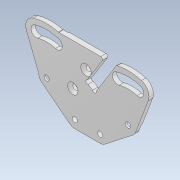
# Autodesk Inventor part: 脚中間フレーム外側
Saved by Autodesk Inventor 2020.2 (Build 242310000, 310)
## iProperties
Created: 2020-03-12
Part Number: 脚中間フレーム外側
Material: アルミニウム 2014-T4
Document SubType Name: Modeling
Designer: aoyam
Density: 2.8 g/cm^3
Appearance: サテン
Mass: 9.40624 g
Surface Area: 56.2254 cm^2
Volume: 3.35937 cm^3
Author: aoyam
Autodesk Inventor part; units mm, degrees
ref_plane "YZ Plane" through (0, 0, 0) normal (1, 0, 0) x (0, 1, 0)
ref_plane "XZ Plane" through (0, 0, 0) normal (0, 1, 0) x (-1, 0, 0)
ref_plane "XY Plane" through (0, 0, 0) normal (0, 0, 1) x (1, 0, 0)
sketch "スケッチ1" plane through (0, 0, 0) normal (0, 0, 1) x (1, 0, 0)
  circle A0 centre (-23.2, 0) radius 14.1 construction
  circle A1 centre (0, 0) radius 9.1 construction
  circle A2 centre (23.2, 0) radius 14.1 construction
  circle A3 centre (-23.2, 0) radius 1.5
  circle A4 centre (-23.2, 0) radius 4.5
  line L0 (0, 0) -> (0, 20.5296)
  line L1 (-47.939, 0) -> (0, 0)
  line L2 (0, 0) -> (0, -20)
  circle A5 centre (0, 15.5) radius 1.5
  circle A6 centre (0, 15.5) radius 4.5 construction
  circle A7 centre (0, 0) radius 11 construction
  line L3 (-38, 31) -> (38, 31)
  line L4 (38, 31) -> (38, -20)
  line L5 (38, -20) -> (-38, -20)
  line L6 (-38, -20) -> (-38, 31)
  circle A8 centre (23.2, 0) radius 4.5
  circle A9 centre (23.2, 0) radius 1.5
  arc A10 (1.5, -5.8095) -> (4.2038, 4.2812) centre (0, 0) ccw
  line L7 (-1.5, -5.8095) -> (-1.5, -11.2574)
  line L8 (1.5, -11.2574) -> (1.5, -5.8095)
  arc A11 (1.6057, 5.7812) -> (-1.6057, 5.7812) centre (0, 0) ccw
  circle A12 centre (0, 0) radius 4
  arc A13 (-4.2038, 4.2812) -> (-1.5, -5.8095) centre (0, 0) ccw
  line L9 (4.2038, 4.2812) -> (7.2283, 9.5198)
  arc A14 (7.2283, 9.5198) -> (4.6302, 11.0198) centre (7.2283, 12.5198) ccw
  line L10 (4.6302, 11.0198) -> (1.6057, 5.7812)
  line L11 (-1.6057, 5.7812) -> (-4.6302, 11.0198)
  arc A15 (-4.6302, 11.0198) -> (-7.2283, 9.5198) centre (-7.2283, 12.5198) ccw
  line L12 (-7.2283, 9.5198) -> (-4.2038, 4.2812)
  circle A16 centre (-7.2283, 12.5198) radius 1.5
  circle A17 centre (7.2283, 12.5198) radius 1.5
  circle A18 centre (-7.2283, -12.5198) radius 1.5
  circle A19 centre (7.2283, -12.5198) radius 1.5
  circle A20 centre (-7.2283, -12.5198) radius 4.5
  circle A21 centre (7.2283, -12.5198) radius 4.5
  line L13 (-25.9762, -3.5416) -> (-10.0045, -16.0614)
  line L14 (-7.2283, -17.0198) -> (7.2283, -17.0198)
  line L15 (10.0045, -16.0614) -> (25.9762, -3.5416)
  line L16 (23.2, 0) -> (38, 0)
  circle A22 centre (7.2283, -12.5198) radius 1.5
  circle A23 centre (-7.2283, -12.5198) radius 1.5
  arc A24 (-18.134, 17.0975) -> (-28.266, 17.0975) centre (-23.2, 0) ccw
  arc A25 (-29.9847, 22.8983) -> (-28.266, 17.0975) centre (-29.1254, 19.9979) ccw
  arc A26 (-16.4153, 22.8983) -> (-29.9847, 22.8983) centre (-23.2, 0) ccw
  arc A27 (-18.134, 17.0975) -> (-16.4153, 22.8983) centre (-17.2746, 19.9979) ccw
  circle A28 centre (0, 15.5) radius 1.5
  arc A29 (28.266, 17.0975) -> (18.134, 17.0975) centre (23.2, 0) ccw
  arc A30 (16.4153, 22.8983) -> (18.134, 17.0975) centre (17.2746, 19.9979) ccw
  arc A31 (29.9847, 22.8983) -> (16.4153, 22.8983) centre (23.2, 0) ccw
  arc A32 (28.266, 17.0975) -> (29.9847, 22.8983) centre (29.1254, 19.9979) ccw
  line L17 (-34, 26) -> (34, 26)
  line L18 (-29.1254, 19.9979) -> (-23.2, 0)
  line L19 (-23.2, 0) -> (-17.2746, 19.9979)
  circle A33 centre (-9.2601, 26) radius 1.25
  circle A34 centre (-23.2, 0) radius 4.5
  circle A35 centre (23.2, 0) radius 4.5
  arc A36 (-18.9863, 14.2211) -> (-27.4137, 14.2211) centre (-23.2, 0) ccw
  arc A37 (-18.9863, 14.2211) -> (-15.563, 25.7747) centre (-17.2746, 19.9979) ccw
  arc A38 (-15.563, 25.7747) -> (-30.837, 25.7747) centre (-23.2, 0) ccw
  arc A39 (-30.837, 25.7747) -> (-27.4137, 14.2211) centre (-29.1254, 19.9979) ccw
  circle A40 centre (-9.2601, 26) radius 4.25
  arc A41 (27.4137, 14.2211) -> (18.9863, 14.2211) centre (23.2, 0) ccw
  arc A42 (27.4137, 14.2211) -> (30.837, 25.7747) centre (29.1254, 19.9979) ccw
  arc A43 (30.837, 25.7747) -> (15.563, 25.7747) centre (23.2, 0) ccw
  arc A44 (15.563, 25.7747) -> (18.9863, 14.2211) centre (17.2746, 19.9979) ccw
  line L20 (-27.7, 0) -> (-34.7286, 17.7833)
  line L21 (-23.2, 26.8823) -> (-10.295, 30.1221)
  line L22 (-8.2253, 30.1221) -> (23.2, 26.8823)
  line L23 (34.9021, 18.2863) -> (27.4137, -1.5794)
  point P0 (-27.7, 0)
  point P1 (27.7, 0)
  point P2 (-38, 0)
  point P3 (28.0091, 0)
  point P4 (34.5946, 17.4704)
  point P5 (-27.7, 0)
  point P6 (27.4137, -1.5794)
  point P7 (16.3694, 26)
  point P8 (-16.3694, 26)
  dimension "d55" = 9
  dimension "d56" = 9
  dimension "d0" = 28.2
  dimension "d1" = 28.2
  dimension "d2" = 18.2
  dimension "d3" = 3
  dimension "d4" = 3
  dimension "d5" = 3
  dimension "d6" = 3
  dimension "d7" = 22
  dimension "d8" = 38
  dimension "d11" = 31
  dimension "d14" = 20
  dimension "d15" = 3
  dimension "d16" = 3
  dimension "d17" = 38
  dimension "d44" = 3
  dimension "d45" = 3
  dimension "d51" = 33.009
  dimension "d52" = 2.5
  dimension "d53" = 14
  dimension "d54" = 10.5
  dimension "d57" = 3
  dimension "d58" = 3
  dimension "d59" = 3
  constraints: 52 point on circle, 48 end point, 41 centre point, 8 tangent, 6 coincident, 5 horizontal, 4 point on line, 3 symmetric about line, 3 vertical, 2 parallel, 2 perpendicular, 1 horizontal alignment, 46 other
  measures "d0" diameter of A2
  measures "d1" diameter of A0
  measures "d2" diameter of A1
  measures "d3" diameter of A3
  measures "d4" diameter of A3
  measures "d5" diameter of A5
  measures "d6" radial gap between concentric circles of A5 A6
  measures "d7" diameter of A7
  measures "d8" distance between parallel lines of L6 L0
  measures "d11" distance between parallel lines of L1 L3
  measures "d14" distance between parallel lines of L5 L1
  measures "d15" diameter of A16
  measures "d16" diameter of A17
  measures "d17" distance between parallel lines of L4 L0
  measures "d44" radial gap between concentric circles of A20 A18
  measures "d45" radial gap between concentric circles of A19 A21
  measures "d51" angle of L19 L18
  measures "d52" diameter of A33
  measures "d53" distance of A28.centre A33.centre
  measures "d54" distance from line of A28.centre L17
  measures "d57" radial gap between concentric circles of A24 A36
  measures "d58" radial gap between concentric circles of A33 A40
  measures "d59" radial gap between concentric circles of A30 A44
extrude "押し出し1" add sketch "スケッチ1" along normal blind 3 contours L1 A4 A3 | A3 L19 A4 L1 | A3 L18 A4 L19 | L1 A4 L18 A3 | L1 A12 L2 L14 A20 L13 A4 | A4 L19 A37 A40 L17 A43 A44 A41 A42 L23 L16 A8 L15 A21 L14 L2 A12 L0 A11 L11 A15 L12 A13 L1 | A4 L18 A36 L19 | L20 A39 L18 A4 | A13 L12 A15 L11 A11 L0 A12 L1 | A36 L18 A24 L19 | L19 A27 A26 A25 L18 A39 A38 L17 A37 A40 | A20 | A12 L0 L1 | L1 L2 A12 | A40 A37 | A37 A40 L17 A33 | L0 A12 L2 | A37 A38 L17 A40 | A38 L17 | A33 L17 | A43 L17 | L17 A43 A42 L23 A41 A44 | A21 | L23 A8 L16 | A8 | L23 A42 | A5 L0 | L0 A5 | A16 | A17 picked at (-9.1528, 25.1164)
sketch "スケッチ3" plane through (0, 0, 3) normal (0, 0, 1) x (1, 0, 0)
  circle A0 centre (7.2283, -12.5198) radius 1.5
  circle A1 centre (-7.2283, -12.5198) radius 1.5
  arc A2 (-18.134, 17.0975) -> (-28.266, 17.0975) centre (-23.2, 0) ccw
  arc A3 (-29.9847, 22.8983) -> (-28.266, 17.0975) centre (-29.1254, 19.9979) ccw
  arc A4 (-16.4153, 22.8983) -> (-29.9847, 22.8983) centre (-23.2, 0) ccw
  arc A5 (-18.134, 17.0975) -> (-16.4153, 22.8983) centre (-17.2746, 19.9979) ccw
  circle A6 centre (0, 15.5) radius 1.5
  arc A7 (28.266, 17.0975) -> (18.134, 17.0975) centre (23.2, 0) ccw
  arc A8 (16.4153, 22.8983) -> (18.134, 17.0975) centre (17.2746, 19.9979) ccw
  arc A9 (29.9847, 22.8983) -> (16.4153, 22.8983) centre (23.2, 0) ccw
  arc A10 (28.266, 17.0975) -> (29.9847, 22.8983) centre (29.1254, 19.9979) ccw
  line L0 (-34, 26) -> (34, 26)
  line L1 (-29.1254, 19.9979) -> (-23.2, 0)
  line L2 (-23.2, 0) -> (-17.2746, 19.9979)
  circle A11 centre (-9.2601, 26) radius 1.25
  circle A12 centre (-23.2, 0) radius 4.5
  circle A13 centre (23.2, 0) radius 4.5
  arc A14 (-18.9863, 14.2211) -> (-27.4137, 14.2211) centre (-23.2, 0) ccw
  arc A15 (-18.9863, 14.2211) -> (-15.563, 25.7747) centre (-17.2746, 19.9979) ccw
  arc A16 (-15.563, 25.7747) -> (-30.837, 25.7747) centre (-23.2, 0) ccw
  arc A17 (-30.837, 25.7747) -> (-27.4137, 14.2211) centre (-29.1254, 19.9979) ccw
  circle A18 centre (-9.2601, 26) radius 4.25
  arc A19 (27.4137, 14.2211) -> (18.9863, 14.2211) centre (23.2, 0) ccw
  arc A20 (27.4137, 14.2211) -> (30.837, 25.7747) centre (29.1254, 19.9979) ccw
  arc A21 (30.837, 25.7747) -> (15.563, 25.7747) centre (23.2, 0) ccw
  arc A22 (15.563, 25.7747) -> (18.9863, 14.2211) centre (17.2746, 19.9979) ccw
  line L3 (-27.7, 0) -> (-34.7286, 17.7833)
  line L4 (-23.2, 26.8823) -> (-10.295, 30.1221)
  line L5 (-8.2253, 30.1221) -> (23.2, 26.8823)
  line L6 (34.9021, 18.2863) -> (27.4137, -1.5794)
  point P0 (0, 0)
  point P1 (0, 0)
  dimension "d46" = 9
  dimension "d47" = 9
  dimension "d38" = 33.009
  dimension "d39" = 2.5
  dimension "d40" = 14
  dimension "d41" = 10.5
  dimension "d48" = 3
  dimension "d49" = 3
  dimension "d50" = 3
  constraints: 38 point on circle, 21 centre point, 14 end point, 2 tangent, 1 coincident, 1 horizontal, 1 horizontal alignment, 1 point on line, 32 other
  measures "d38" angle of L2 L1
  measures "d39" diameter of A11
  measures "d40" distance of A6.centre A11.centre
  measures "d41" distance from line of A6.centre L0
  measures "d48" radial gap between concentric circles of A2 A14
  measures "d49" radial gap between concentric circles of A11 A18
  measures "d50" radial gap between concentric circles of A8 A22
sketch "スケッチ5" plane through (0, 0, 0) normal (0, 0, -1) x (-1, 0, 0)
  circle A0 centre (-23.2, 0) radius 1.5 projected
  circle A1 centre (23.2, 0) radius 1.5 projected
  circle A2 centre (-23.2, 0) radius 3
  circle A3 centre (23.2, 0) radius 3
  point P0 (0, 0)
  dimension "d25" = 6
  dimension "d26" = 6
  constraints: 2 centre point, 2 coincident
  measures "d25" diameter of A2
  measures "d26" diameter of A3
extrude "押し出し4" cut sketch "スケッチ5" against normal blind 2
sketch "スケッチ6" plane through (0, 0, 0) normal (0, 0, -1) x (-1, 0, 0)
  circle A0 centre (-7.2283, -12.5198) radius 1.5 projected
  circle A1 centre (7.2283, -12.5198) radius 1.5 projected
  circle A2 centre (-7.2283, -12.5198) radius 3
  circle A3 centre (7.2283, -12.5198) radius 3
  point P0 (0, 0)
  dimension "d32" = 6
  dimension "d33" = 6
  constraints: 2 centre point, 2 coincident
  measures "d32" diameter of A2
  measures "d33" diameter of A3
extrude "押し出し5" cut sketch "スケッチ6" against normal blind 0.5
sketch "スケッチ9" plane through (0, 0, 3) normal (0, 0, 1) x (1, 0, 0)
  line L0 (27.4137, -1.5794) -> (34.5946, 17.4704) projected
  arc A0 (34.5946, 17.4704) -> (30.837, 25.7747) centre (29.1254, 19.9979) ccw projected
  arc A1 (30.837, 25.7747) -> (16.3694, 26) centre (23.2, 0) ccw projected
  arc A2 (-16.3694, 26) -> (-30.837, 25.7747) centre (-23.2, 0) ccw projected
  arc A3 (-30.837, 25.7747) -> (-34.7286, 17.7833) centre (-29.1254, 19.9979) ccw projected
  line L1 (-34.7286, 17.7833) -> (-27.7, 0) projected
  arc A4 (-27.7, 0) -> (-25.9762, -3.5416) centre (-23.2, 0) ccw projected
  line L2 (-25.9762, -3.5416) -> (-10.0045, -16.0614) projected
  arc A5 (-10.0045, -16.0614) -> (-7.2283, -17.0198) centre (-7.2283, -12.5198) ccw projected
  line L3 (-7.2283, -17.0198) -> (7.2283, -17.0198) projected
  arc A6 (7.2283, -17.0198) -> (10.0045, -16.0614) centre (7.2283, -12.5198) ccw projected
  line L4 (10.0045, -16.0614) -> (25.9762, -3.5416) projected
  arc A7 (25.9762, -3.5416) -> (27.4137, -1.5794) centre (23.2, 0) ccw projected
  circle A8 centre (-7.2283, -12.5198) radius 1.5 projected
  circle A9 centre (23.2, 0) radius 1.5 projected
  circle A10 centre (-23.2, 0) radius 1.5 projected
  circle A11 centre (7.2283, -12.5198) radius 1.5 projected
  arc A12 (28.266, 17.0975) -> (29.9847, 22.8983) centre (29.1254, 19.9979) ccw projected
  arc A13 (28.266, 17.0975) -> (18.134, 17.0975) centre (23.2, 0) ccw projected
  arc A14 (16.4153, 22.8983) -> (18.134, 17.0975) centre (17.2746, 19.9979) ccw projected
  arc A15 (29.9847, 22.8983) -> (16.4153, 22.8983) centre (23.2, 0) ccw projected
  arc A16 (-29.9847, 22.8983) -> (-28.266, 17.0975) centre (-29.1254, 19.9979) ccw projected
  arc A17 (-16.4153, 22.8983) -> (-29.9847, 22.8983) centre (-23.2, 0) ccw projected
  arc A18 (-18.134, 17.0975) -> (-16.4153, 22.8983) centre (-17.2746, 19.9979) ccw projected
  arc A19 (-18.134, 17.0975) -> (-28.266, 17.0975) centre (-23.2, 0) ccw projected
  line L5 (16.3694, 26) -> (-16.3694, 26) projected
  point P0 (0, 0)
sketch "翼" plane through (0, 0, 3) normal (0, 0, 1) x (1, 0, 0)
  arc A0 (-18.1381, 17.1031) -> (-16.4194, 22.9038) centre (-17.2788, 20.0034) ccw
  arc A1 (28.2619, 17.1031) -> (29.9806, 22.9038) centre (29.1212, 20.0034) ccw
  line L0 (27.4137, -1.5794) -> (34.5946, 17.4704) projected
  arc A2 (34.5946, 17.4704) -> (30.837, 25.7747) centre (29.1254, 19.9979) ccw projected
  arc A3 (30.837, 25.7747) -> (16.3694, 26) centre (23.2, 0) ccw projected
  line L1 (16.3694, 26) -> (-16.3694, 26) projected
  arc A4 (-16.3694, 26) -> (-30.837, 25.7747) centre (-23.2, 0) ccw projected
  arc A5 (-30.837, 25.7747) -> (-34.7286, 17.7833) centre (-29.1254, 19.9979) ccw projected
  line L2 (-34.7286, 17.7833) -> (-27.7, 0) projected
  arc A6 (-27.7, 0) -> (-25.9762, -3.5416) centre (-23.2, 0) ccw projected
  line L3 (-25.9762, -3.5416) -> (-10.0045, -16.0614) projected
  arc A7 (-10.0045, -16.0614) -> (-7.2283, -17.0198) centre (-7.2283, -12.5198) ccw projected
  line L4 (-7.2283, -17.0198) -> (7.2283, -17.0198) projected
  arc A8 (7.2283, -17.0198) -> (10.0045, -16.0614) centre (7.2283, -12.5198) ccw projected
  line L5 (10.0045, -16.0614) -> (25.9762, -3.5416) projected
  arc A9 (25.9762, -3.5416) -> (27.4137, -1.5794) centre (23.2, 0) ccw projected
  arc A10 (28.266, 17.0975) -> (18.134, 17.0975) centre (23.2, 0) ccw projected
  arc A11 (16.4153, 22.8983) -> (18.134, 17.0975) centre (17.2746, 19.9979) ccw projected
  arc A12 (29.9847, 22.8983) -> (16.4153, 22.8983) centre (23.2, 0) ccw projected
  arc A13 (28.266, 17.0975) -> (29.9847, 22.8983) centre (29.1254, 19.9979) ccw projected
  arc A14 (-29.9847, 22.8983) -> (-28.266, 17.0975) centre (-29.1254, 19.9979) ccw projected
  arc A15 (-16.4153, 22.8983) -> (-29.9847, 22.8983) centre (-23.2, 0) ccw projected
  arc A16 (-18.134, 17.0975) -> (-16.4153, 22.8983) centre (-17.2746, 19.9979) ccw projected
  arc A17 (-18.134, 17.0975) -> (-28.266, 17.0975) centre (-23.2, 0) ccw projected
  circle A18 centre (-23.2, 0) radius 1.5 projected
  circle A19 centre (7.2283, -12.5198) radius 1.5 projected
  circle A20 centre (23.2, 0) radius 1.5 projected
  circle A21 centre (-7.2283, -12.5198) radius 1.5 projected
  line L6 (0.0889, 10.0467) -> (15.7158, 35.055)
  line L7 (15.7158, 35.055) -> (19.9561, 32.4054)
  line L8 (19.9561, 32.4054) -> (4.3292, 7.3971)
  line L9 (4.3292, 7.3971) -> (0.0889, 10.0467)
  line L10 (15.5568, 35.744) -> (-0.865, 9.4636)
  line L11 (-0.865, 9.4636) -> (4.2233, 6.2841)
  line L12 (4.2233, 6.2841) -> (20.6451, 32.5644)
  line L13 (20.6451, 32.5644) -> (15.5568, 35.744)
  line L14 (-11.2804, 3.1744) -> (-0.2027, 20.9024)
  circle A22 centre (-0.7595, 15.2936) radius 1.5
  circle A23 centre (-8.2799, 2.315) radius 1.5
  circle A24 centre (0.1581, 9.6998) radius 1.05
  circle A25 centre (3.9871, 7.3072) radius 1.05
  line L15 (0.1581, 9.6998) -> (-0.865, 9.4636)
  line L16 (4.2233, 6.2841) -> (3.9871, 7.3072)
  point P0 (0, 0)
  point P1 (4.3292, 7.3971)
  point P2 (0.3943, 8.6767)
  point P3 (-0.0781, 10.7229)
  point P4 (5.0102, 7.5434)
  point P5 (2.964, 7.071)
  dimension "d279" = 2.1
  dimension "d280" = 2.1
  dimension "d250" = 5
  dimension "d251" = 58
  dimension "d252" = 0.5
  dimension "d253" = 6
  dimension "d254" = 3
  dimension "d255" = 3
  dimension "d256" = 3
  dimension "d257" = 3
  dimension "d258" = 15
  dimension "d259" = 4
  dimension "d277" = 0.5
  dimension "d278" = 1
  dimension "d282" = 45
  dimension "d283" = 45
  constraints: 22 end point, 4 centre point, 4 point on circle, 2 parallel, 2 perpendicular, 1 coincident, 17 other
  measures "d250" distance between parallel lines of L8 L6
  measures "d251" angle of L1 L8
  measures "d252" distance between parallel lines of L6 L10
  measures "d253" distance between parallel lines of L14 L6
  measures "d254" diameter of A22
  measures "d255" diameter of A23
  measures "d256" distance from line of L10 A22.centre
  measures "d257" distance from line of L14 A23.centre
  measures "d258" distance of A22.centre A23.centre
  measures "d259" distance from line of L9 A22.centre
  measures "d277" distance between parallel lines of L12 L8
  measures "d278" distance between parallel lines of L11 L9
  measures "d282" angle of L15 L10
  measures "d283" angle of L11 L16
extrude "押し出し13" cut sketch "翼" against normal blind 10 contours L12 A25 L8 L1 A3 | A3 L1 L8 L7 L6 L10 L13 L12 | A25 L12 | L12 L11 A25 L9 L8 | L8 A25 L9 A24 L6 L1 | L1 L6 L7 L8 | A25 L11 | L8 L9 A25 | L6 A24 L10 L1 | L11 A24 L9 A25 | A24 L9 L6 | L6 L9 A24 L11 L10 | A24 L11 | L10 A24 | A22 | A23
sketch "スケッチ10" plane through (0, 0, 0) normal (0, 0, -1) x (-1, 0, 0)
  arc A0 (-11.2521, 18.8307) -> (-13.5147, 24.8231) centre (-17.1301, 20.0347) ccw
  line L0 (-31.1595, 38.1455) -> (-13.5147, 24.8231)
  line L1 (-11.2521, 18.8307) -> (-15.418, -1.5082)
  arc A1 (-25.2739, -7.6441) -> (-15.418, -1.5082) centre (-23.2553, 0.0971) ccw
  arc A2 (-16.4706, 22.9953) -> (-30.04, 22.9953) centre (-23.2553, 0.0971) ccw
  arc A3 (-30.04, 22.9953) -> (-28.3213, 17.1946) centre (-29.1807, 20.095) ccw
  arc A4 (-18.1893, 17.1946) -> (-28.3213, 17.1946) centre (-23.2553, 0.0971) ccw
  arc A5 (-18.1893, 17.1946) -> (-16.4706, 22.9953) centre (-17.3299, 20.095) ccw
  line L2 (-30.5569, 38.9436) -> (-12.9121, 25.6211)
  arc A6 (-10.2725, 18.6301) -> (-12.9121, 25.6211) centre (-17.1301, 20.0347) ccw
  line L3 (-10.2725, 18.6301) -> (-14.4383, -1.7088)
  arc A7 (-25.5262, -8.6117) -> (-14.4383, -1.7088) centre (-23.2553, 0.0971) ccw
  circle A8 centre (-7.2283, -12.5198) radius 3 projected
  line L4 (-27.4137, -1.5794) -> (-34.5946, 17.4704) projected
  line L5 (-10.0045, -16.0614) -> (-25.9762, -3.5416) projected
  arc A9 (-10.0045, -16.0614) -> (-7.2283, -17.0198) centre (-7.2283, -12.5198) ccw projected
  line L6 (7.2283, -17.0198) -> (-7.2283, -17.0198) projected
  line L7 (25.9762, -3.5416) -> (10.0045, -16.0614) projected
  line L8 (34.7286, 17.7833) -> (27.7, 0) projected
  arc A10 (34.7286, 17.7833) -> (30.837, 25.7747) centre (29.1254, 19.9979) ccw projected
  arc A11 (30.837, 25.7747) -> (16.3694, 26) centre (23.2, 0) ccw projected
  line L9 (-9.6042, 26) -> (16.3694, 26) projected
  arc A12 (-16.7719, 26.1024) -> (-30.837, 25.7747) centre (-23.2, 0) ccw projected
  arc A13 (-30.837, 25.7747) -> (-34.5946, 17.4704) centre (-29.1254, 19.9979) ccw projected
  arc A14 (-18.134, 17.0975) -> (-28.266, 17.0975) centre (-23.2, 0) ccw projected
  arc A15 (-29.9847, 22.8983) -> (-28.266, 17.0975) centre (-29.1254, 19.9979) ccw projected
  arc A16 (-16.4153, 22.8983) -> (-29.9847, 22.8983) centre (-23.2, 0) ccw projected
  arc A17 (-18.134, 17.0975) -> (-16.4153, 22.8983) centre (-17.2746, 19.9979) ccw projected
  arc A18 (28.266, 17.0975) -> (29.9847, 22.8983) centre (29.1254, 19.9979) ccw projected
  arc A19 (28.266, 17.0975) -> (18.134, 17.0975) centre (23.2, 0) ccw projected
  arc A20 (16.4153, 22.8983) -> (18.134, 17.0975) centre (17.2746, 19.9979) ccw projected
  arc A21 (29.9847, 22.8983) -> (16.4153, 22.8983) centre (23.2, 0) ccw projected
  line L10 (3.3826, 0) -> (3.3826, 26)
  line L11 (37.3221, 38.9436) -> (19.6773, 25.6211)
  arc A22 (19.6773, 25.6211) -> (17.0377, 18.6301) centre (23.8953, 20.0347) ccw
  line L12 (17.0377, 18.6301) -> (21.2036, -1.7088)
  arc A23 (21.2036, -1.7088) -> (32.2915, -8.6117) centre (30.0205, 0.0971) ccw
  arc A24 (-27.4137, -1.5794) -> (-25.9762, -3.5416) centre (-23.2, 0) ccw projected
  arc A25 (7.2283, -17.0198) -> (10.0045, -16.0614) centre (7.2283, -12.5198) ccw projected
  arc A26 (25.9762, -3.5416) -> (27.7, 0) centre (23.2, 0) ccw projected
  line L13 (-0.6699, 9.1236) -> (-3.2296, 7.5019) projected
  line L14 (-5.2787, 7.9615) -> (-16.7719, 26.1024) projected
  line L15 (-9.6042, 26) -> (-0.2103, 11.1726) projected
  arc A27 (-0.6699, 9.1236) -> (-0.2103, 11.1726) centre (-0.4401, 10.1481) ccw projected
  arc A28 (-5.2787, 7.9615) -> (-3.2296, 7.5019) centre (-4.2541, 7.7317) ccw projected
  point P0 (13.4139, 26)
  point P1 (23.1707, -5.7407)
  point P2 (-19.9427, -8.2711)
  point P3 (-13.4139, 26)
  point P4 (-31.781, 18.5494)
  point P5 (-14.6743, 21.5435)
  point P6 (21.2542, 26.8118)
  point P7 (-10.7037, 16.5244)
  point P8 (17.3768, 16.9746)
  point P9 (17.6686, 23.2329)
  dimension "d177" = 1
  constraints: 20 point on circle, 14 end point, 10 centre point, 7 symmetric about line, 1 midpoint, 9 other
  measures "d177" distance between parallel lines of L0 L2
sketch "スケッチ13" plane through (0, 0, 0.5) normal (0, 0, -1) x (-1, 0, 0)
  circle A0 centre (-7.2283, -12.5198) radius 1.5 projected
  circle A1 centre (7.2283, -12.5198) radius 1.5 projected
  arc A2 (30.1268, 23.3777) -> (16.7004, 23.5) centre (23.2, 0) ccw
  arc A3 (32.4036, 18.7022) -> (30.1268, 23.3777) centre (29.1254, 19.9979) ccw
  line L0 (32.4036, 18.7022) -> (27.8387, 7.1525)
  arc A4 (27.8387, 7.1525) -> (17.9117, -6.6865) centre (23.2, 0) ccw
  line L1 (17.9117, -6.6865) -> (8.4622, -14.0938)
  arc A5 (7.2283, -14.5198) -> (8.4622, -14.0938) centre (7.2283, -12.5198) ccw
  line L2 (7.2283, -14.5198) -> (-7.2283, -14.5198)
  arc A6 (-8.4622, -14.0938) -> (-7.2283, -14.5198) centre (-7.2283, -12.5198) ccw
  line L3 (-8.4622, -14.0938) -> (-17.9117, -6.6865)
  arc A7 (-17.9117, -6.6865) -> (-27.9945, 7.049) centre (-23.2, 0) ccw
  line L4 (-27.9945, 7.049) -> (-32.2915, 18.4482)
  arc A8 (-30.1268, 23.3777) -> (-32.2915, 18.4482) centre (-29.1254, 19.9979) ccw
  arc A9 (-18.3304, 23.8911) -> (-30.1268, 23.3777) centre (-23.2, 0) ccw
  line L5 (-18.3304, 23.8911) -> (-5.2578, 3.2573)
  line L6 (-5.2578, 3.2573) -> (4.0342, 9.1444)
  line L7 (4.0342, 9.1444) -> (-5.0608, 23.5)
  line L8 (-5.0608, 23.5) -> (16.7004, 23.5)
  line L9 (-23.2, 0) -> (-9.8054, 10.4352) construction
  line L10 (-22.4318, -0.9861) -> (-9.0372, 9.4491)
  line L11 (-10.5736, 11.4212) -> (-23.9682, 0.9861)
  arc A10 (-23.9682, 0.9861) -> (-22.4318, -0.9861) centre (-23.2, 0) ccw
  arc A11 (-9.0372, 9.4491) -> (-10.5736, 11.4212) centre (-9.8054, 10.4352) ccw
  line L12 (-7.2283, -12.5198) -> (-5.2578, 3.2573) construction
  line L13 (-5.9879, -12.6747) -> (-4.0175, 3.1024)
  line L14 (-6.4982, 3.4123) -> (-8.4687, -12.3649)
  arc A12 (-8.4687, -12.3649) -> (-5.9879, -12.6747) centre (-7.2283, -12.5198) ccw
  arc A13 (-4.0175, 3.1024) -> (-6.4982, 3.4123) centre (-5.2578, 3.2573) ccw
  line L15 (4.0342, 9.1444) -> (23.2, 0) construction
  line L16 (3.496, 8.0162) -> (22.6617, -1.1282)
  line L17 (23.7383, 1.1282) -> (4.5725, 10.2726)
  arc A14 (4.5725, 10.2726) -> (3.496, 8.0162) centre (4.0342, 9.1444) ccw
  arc A15 (22.6617, -1.1282) -> (23.7383, 1.1282) centre (23.2, 0) ccw
  line L18 (17.2746, 19.9979) -> (4.0342, 9.1444) construction
  line L19 (16.4822, 20.9646) -> (3.2418, 10.1111)
  line L20 (4.8267, 8.1777) -> (18.0671, 19.0312)
  arc A16 (18.0671, 19.0312) -> (16.4822, 20.9646) centre (17.2746, 19.9979) ccw
  arc A17 (3.2418, 10.1111) -> (4.8267, 8.1777) centre (4.0342, 9.1444) ccw
  line L21 (7.2283, -12.6747) -> (0.2333, 6.7363) construction
  line L22 (8.4043, -12.2509) -> (1.4092, 7.16)
  line L23 (-0.9427, 6.3125) -> (6.0523, -13.0985)
  arc A18 (6.0523, -13.0985) -> (8.4043, -12.2509) centre (7.2283, -12.6747) ccw
  arc A19 (1.4092, 7.16) -> (-0.9427, 6.3125) centre (0.2333, 6.7363) ccw
  circle A20 centre (-7.2283, -12.5198) radius 4
  circle A21 centre (7.2283, -12.5198) radius 4
  arc A22 (-30.695, 25.2953) -> (-27.5558, 14.7005) centre (-29.1254, 19.9979) ccw
  arc A23 (-15.705, 25.2953) -> (-30.695, 25.2953) centre (-23.2, 0) ccw
  arc A24 (-18.8442, 14.7005) -> (-15.705, 25.2953) centre (-17.2746, 19.9979) ccw
  arc A25 (-18.8442, 14.7005) -> (-27.5558, 14.7005) centre (-23.2, 0) ccw
  arc A26 (27.5558, 14.7005) -> (18.8442, 14.7005) centre (23.2, 0) ccw
  arc A27 (27.5558, 14.7005) -> (30.695, 25.2953) centre (29.1254, 19.9979) ccw
  arc A28 (30.695, 25.2953) -> (15.705, 25.2953) centre (23.2, 0) ccw
  arc A29 (15.705, 25.2953) -> (18.8442, 14.7005) centre (17.2746, 19.9979) ccw
  point P0 (0, 0)
  point P1 (-16.5027, 5.2176)
  point P2 (-6.2431, -4.6312)
  point P3 (13.6171, 4.5722)
  point P4 (10.6544, 14.5711)
  point P5 (3.7308, -2.9692)
  point P6 (12.3201, 17.5528)
  point P7 (13.0014, 23.5)
  point P8 (3.3603, 10.2082)
  point P9 (13.905, 15.6194)
  point P10 (6.3485, 9.4252)
  point P11 (16.1273, 4.7595)
  point P12 (30.8398, 14.7456)
  point P13 (7.061, -8.5233)
  point P14 (11.1885, -11.9567)
  point P15 (15.0508, 2.5032)
  point P16 (2.9783, 8.4754)
  point P17 (1.2892, 7.4052)
  point P18 (3.7642, -14.5198)
  point P19 (4.7207, -9.4034)
  point P20 (-0.8485, 6.0509)
  point P21 (-4.2019, 3.9263)
  point P22 (-5.517, -8.9043)
  point P23 (-3.7642, -14.5198)
  point P24 (-11.1885, -11.9567)
  point P25 (-7.9978, -8.5945)
  point P26 (-5.9268, 4.3133)
  point P27 (-9.1332, 9.3742)
  point P28 (-15.7794, 4.1965)
  point P29 (-30.9038, 14.767)
  point P30 (-17.3158, 6.1686)
  point P31 (-10.4743, 11.4911)
  point P32 (-13.3807, 16.0784)
  dimension "d189" = 2.5
  dimension "d190" = 2.5
  dimension "d191" = 2.5
  dimension "d192" = 2.5
  dimension "d193" = 2.5
  dimension "d194" = 2.5
  dimension "d195" = 2.5
  constraints: 58 end point, 52 point on circle, 28 centre point, 20 tangent, 5 midpoint, 5 parallel, 2 point on line
  measures "d189" diameter of A11
  measures "d190" diameter of A13
  measures "d191" diameter of A15
  measures "d192" diameter of A17
  measures "d193" diameter of A19
  measures "d194" radial gap between concentric circles of A0 A20
  measures "d195" radial gap between concentric circles of A1 A21
sketch "スケッチ20" plane through (0, 0, 0) normal (0, 0, -1) x (-1, 0, 0)
  arc A0 (28.266, 17.0975) -> (29.9847, 22.8983) centre (29.1254, 19.9979) ccw projected
  arc A1 (28.266, 17.0975) -> (18.134, 17.0975) centre (23.2, 0) ccw projected
  arc A2 (16.4153, 22.8983) -> (18.134, 17.0975) centre (17.2746, 19.9979) ccw projected
  arc A3 (29.9847, 22.8983) -> (16.4153, 22.8983) centre (23.2, 0) ccw projected
  arc A4 (-18.134, 17.0975) -> (-28.266, 17.0975) centre (-23.2, 0) ccw projected
  arc A5 (-29.9847, 22.8983) -> (-28.266, 17.0975) centre (-29.1254, 19.9979) ccw projected
  arc A6 (-16.4153, 22.8983) -> (-29.9847, 22.8983) centre (-23.2, 0) ccw projected
  arc A7 (-18.134, 17.0975) -> (-16.4153, 22.8983) centre (-17.2746, 19.9979) ccw projected
  line L0 (-9.4681, 26) -> (0.0781, 10.7229) projected
  line L1 (-0.3943, 8.6767) -> (-2.964, 7.071) projected
  line L2 (-5.0102, 7.5434) -> (-16.5766, 26.0535) projected
  arc A8 (-16.5766, 26.0535) -> (-30.837, 25.7747) centre (-23.2, 0) ccw projected
  arc A9 (-30.837, 25.7747) -> (-34.5946, 17.4704) centre (-29.1254, 19.9979) ccw projected
  line L3 (-27.4137, -1.5794) -> (-34.5946, 17.4704) projected
  arc A10 (-27.4137, -1.5794) -> (-25.9762, -3.5416) centre (-23.2, 0) ccw projected
  line L4 (-10.0045, -16.0614) -> (-25.9762, -3.5416) projected
  arc A11 (-10.0045, -16.0614) -> (-7.2283, -17.0198) centre (-7.2283, -12.5198) ccw projected
  line L5 (7.2283, -17.0198) -> (-7.2283, -17.0198) projected
  arc A12 (7.2283, -17.0198) -> (10.0045, -16.0614) centre (7.2283, -12.5198) ccw projected
  line L6 (25.9762, -3.5416) -> (10.0045, -16.0614) projected
  arc A13 (25.9762, -3.5416) -> (27.7, 0) centre (23.2, 0) ccw projected
  line L7 (34.7286, 17.7833) -> (27.7, 0) projected
  arc A14 (34.7286, 17.7833) -> (30.837, 25.7747) centre (29.1254, 19.9979) ccw projected
  arc A15 (30.837, 25.7747) -> (16.3694, 26) centre (23.2, 0) ccw projected
  line L8 (-9.4681, 26) -> (16.3694, 26) projected
  circle A16 centre (-23.2, 0) radius 3 projected
  circle A17 centre (23.2, 0) radius 3 projected
  circle A18 centre (-7.2283, -12.5198) radius 3 projected
  circle A19 centre (7.2283, -12.5198) radius 3 projected
  circle A20 centre (0.7595, 15.2936) radius 1.5 projected
  circle A21 centre (8.2799, 2.315) radius 1.5 projected
  arc A22 (30.1268, 23.3777) -> (16.7004, 23.5) centre (23.2, 0) ccw
  arc A23 (32.4036, 18.7022) -> (30.1268, 23.3777) centre (29.1254, 19.9979) ccw
  line L9 (32.4036, 18.7022) -> (25.1631, 0.3826)
  arc A24 (24.4339, -1.574) -> (25.1631, 0.3826) centre (23.2, 0) ccw
  line L10 (24.4339, -1.574) -> (8.4622, -14.0938)
  arc A25 (7.2283, -14.5198) -> (8.4622, -14.0938) centre (7.2283, -12.5198) ccw
  line L11 (7.2283, -14.5198) -> (-7.2283, -14.5198)
  arc A26 (-8.4622, -14.0938) -> (-7.2283, -14.5198) centre (-7.2283, -12.5198) ccw
  line L12 (-8.4622, -14.0938) -> (-24.4339, -1.574)
  arc A27 (-25.0714, -0.7054) -> (-24.4339, -1.574) centre (-23.2, 0) ccw
  line L13 (-25.0714, -0.7054) -> (-32.2915, 18.4482)
  arc A28 (-30.1268, 23.3777) -> (-32.2915, 18.4482) centre (-29.1254, 19.9979) ccw
  arc A29 (-18.1498, 23.8535) -> (-30.1268, 23.3777) centre (-23.2, 0) ccw
  line L14 (-18.1498, 23.8535) -> (-5.0186, 2.8392)
  line L15 (-5.0186, 2.8392) -> (4.3099, 8.6683)
  line L16 (4.3099, 8.6683) -> (-4.958, 23.5)
  line L17 (-4.958, 23.5) -> (16.7004, 23.5)
  arc A30 (-18.8442, 14.7005) -> (-27.5558, 14.7005) centre (-23.2, 0) ccw
  arc A31 (-18.8442, 14.7005) -> (-15.705, 25.2953) centre (-17.2746, 19.9979) ccw
  arc A32 (-15.705, 25.2953) -> (-30.695, 25.2953) centre (-23.2, 0) ccw
  arc A33 (-30.695, 25.2953) -> (-27.5558, 14.7005) centre (-29.1254, 19.9979) ccw
  circle A34 centre (-23.2, 0) radius 5.5
  circle A35 centre (-7.2283, -12.5198) radius 5.5
  circle A36 centre (7.2283, -12.5198) radius 5.5
  circle A37 centre (0.7595, 15.2936) radius 4
  circle A38 centre (8.2799, 2.315) radius 4
  circle A39 centre (23.2, 0) radius 5.5
  arc A40 (27.5558, 14.7005) -> (18.8442, 14.7005) centre (23.2, 0) ccw
  arc A41 (27.5558, 14.7005) -> (30.695, 25.2953) centre (29.1254, 19.9979) ccw
  arc A42 (30.695, 25.2953) -> (15.705, 25.2953) centre (23.2, 0) ccw
  arc A43 (15.705, 25.2953) -> (18.8442, 14.7005) centre (17.2746, 19.9979) ccw
  line L18 (-23.2, 0) -> (-13.3259, 16.1336) construction
  line L19 (-22.1338, -0.6525) -> (-12.2597, 15.4811)
  line L20 (-14.392, 16.7861) -> (-24.2662, 0.6525)
  arc A44 (-24.2662, 0.6525) -> (-22.1338, -0.6525) centre (-23.2, 0) ccw
  arc A45 (-12.2597, 15.4811) -> (-14.392, 16.7861) centre (-13.3259, 16.1336) ccw
  line L21 (-5.0186, 2.8392) -> (-7.2283, -12.5198) construction
  line L22 (-6.2559, 3.0172) -> (-8.4656, -12.3418)
  line L23 (-5.991, -12.6978) -> (-3.7814, 2.6612)
  arc A46 (-3.7814, 2.6612) -> (-6.2559, 3.0172) centre (-5.0186, 2.8392) ccw
  arc A47 (-8.4656, -12.3418) -> (-5.991, -12.6978) centre (-7.2283, -12.5198) ccw
  line L24 (8.2799, 2.315) -> (7.2283, -12.5198) construction
  line L25 (7.033, 2.4034) -> (5.9814, -12.4314)
  line L26 (8.4752, -12.6082) -> (9.5268, 2.2266)
  arc A48 (9.5268, 2.2266) -> (7.033, 2.4034) centre (8.2799, 2.315) ccw
  arc A49 (5.9814, -12.4314) -> (8.4752, -12.6082) centre (7.2283, -12.5198) ccw
  line L27 (8.2799, 2.315) -> (23.2, 0) construction
  line L28 (8.0882, 1.0798) -> (23.0083, -1.2352)
  line L29 (23.3917, 1.2352) -> (8.4716, 3.5502)
  arc A50 (8.4716, 3.5502) -> (8.0882, 1.0798) centre (8.2799, 2.315) ccw
  arc A51 (23.0083, -1.2352) -> (23.3917, 1.2352) centre (23.2, 0) ccw
  line L30 (0.7595, 15.2936) -> (8.2799, 2.315) construction
  line L31 (-0.322, 14.6669) -> (7.1983, 1.6883)
  line L32 (9.3614, 2.9417) -> (1.8411, 15.9203)
  arc A52 (1.8411, 15.9203) -> (-0.322, 14.6669) centre (0.7595, 15.2936) ccw
  arc A53 (7.1983, 1.6883) -> (9.3614, 2.9417) centre (8.2799, 2.315) ccw
  line L33 (17.2746, 19.9979) -> (8.2799, 2.315) construction
  line L34 (16.1605, 20.5646) -> (7.1658, 2.8817)
  line L35 (9.394, 1.7483) -> (18.3888, 19.4312)
  arc A54 (18.3888, 19.4312) -> (16.1605, 20.5646) centre (17.2746, 19.9979) ccw
  arc A55 (7.1658, 2.8817) -> (9.394, 1.7483) centre (8.2799, 2.315) ccw
  arc A56 (-0.3943, 8.6767) -> (0.0781, 10.7229) centre (-0.1581, 9.6998) ccw projected
  arc A57 (-5.0102, 7.5434) -> (-2.964, 7.071) centre (-3.9871, 7.3072) ccw projected
  point P0 (0, 0)
  point P1 (-18.2629, 8.0668)
  point P2 (-6.1235, -4.8403)
  point P3 (7.7541, -5.1024)
  point P4 (15.7399, 1.1575)
  point P5 (4.5197, 8.8043)
  point P6 (12.7773, 11.1565)
  point P7 (8.8885, 6.2684)
  point P8 (13.7205, 15.7678)
  point P9 (13.0014, 23.5)
  point P10 (-1.7675, 18.3942)
  point P11 (3.7461, 12.6327)
  point P12 (7.4565, 6.2293)
  point P13 (15.9488, 14.6343)
  point P14 (11.1167, 5.135)
  point P15 (12.2263, 2.9676)
  point P16 (18.0989, 2.0564)
  point P17 (26.6914, 4.2497)
  point P18 (30.8398, 14.7456)
  point P19 (17.7156, -0.414)
  point P20 (11.843, 0.4972)
  point P21 (9.2581, -1.5635)
  point P22 (8.8539, -7.2655)
  point P23 (12.4944, -10.933)
  point P24 (20.4016, -4.7348)
  point P25 (5.2934, 4.9759)
  point P26 (3.4612, 8.1379)
  point P27 (-3.9586, 3.5016)
  point P28 (-5.2283, -7.3963)
  point P29 (-2.1048, -14.5198)
  point P30 (2.1048, -14.5198)
  point P31 (6.3602, -7.0887)
  point P32 (6.7643, -1.3868)
  point P33 (-5.681, 3.8992)
  point P34 (-12.5855, 14.9487)
  point P35 (-19.3379, 3.9159)
  point P36 (-20.4016, -4.7348)
  point P37 (-12.4944, -10.933)
  point P38 (-7.7028, -7.0403)
  point P39 (-30.9038, 14.767)
  point P40 (-26.8786, 4.0887)
  point P41 (-21.4702, 5.2209)
  point P42 (-15.6602, 14.714)
  dimension "d260" = 2.5
  dimension "d261" = 2.5
  dimension "d262" = 2.5
  dimension "d263" = 2.5
  dimension "d264" = 2.5
  dimension "d265" = 2.5
  dimension "d266" = 2.5
  dimension "d267" = 2.5
  dimension "d268" = 2.5
  dimension "d269" = 2.5
  dimension "d270" = 2.5
  dimension "d271" = 2.5
  dimension "d272" = 2.5
  dimension "d273" = 2.5
  dimension "d274" = 2.5
  constraints: 66 end point, 57 point on circle, 34 centre point, 24 tangent, 6 midpoint, 6 parallel, 1 point on line, 22 other
  measures "d260" distance between parallel lines of L8 L17
  measures "d261" radial gap between concentric circles of A4 A30
  measures "d262" radial gap between concentric circles of A16 A34
  measures "d263" radial gap between concentric circles of A18 A35
  measures "d264" radial gap between concentric circles of A19 A36
  measures "d265" radial gap between concentric circles of A20 A37
  measures "d266" radial gap between concentric circles of A21 A38
  measures "d267" radial gap between concentric circles of A17 A39
  measures "d268" radial gap between concentric circles of A2 A43
  measures "d269" diameter of A45
  measures "d270" diameter of A47
  measures "d271" diameter of A49
  measures "d272" diameter of A51
  measures "d273" diameter of A53
  measures "d274" diameter of A55
sketch "スケッチ17" plane through (0, 0, 0) normal (0, 0, -1) x (-1, 0, 0)
  arc A0 (-11.2521, 18.8307) -> (-13.5147, 24.8231) centre (-17.1301, 20.0347) ccw
  line L0 (-31.1595, 38.1455) -> (-13.5147, 24.8231)
  line L1 (-11.2521, 18.8307) -> (-15.418, -1.5082)
  arc A1 (-25.2739, -7.6441) -> (-15.418, -1.5082) centre (-23.2553, 0.0971) ccw
  line L2 (-30.5569, 38.9436) -> (-12.9121, 25.6211)
  arc A2 (-10.2725, 18.6301) -> (-12.9121, 25.6211) centre (-17.1301, 20.0347) ccw
  line L3 (-10.2725, 18.6301) -> (-14.4383, -1.7088)
  arc A3 (-25.5262, -8.6117) -> (-14.4383, -1.7088) centre (-23.2553, 0.0971) ccw
  arc A4 (28.266, 17.0975) -> (29.9847, 22.8983) centre (29.1254, 19.9979) ccw projected
  arc A5 (28.266, 17.0975) -> (18.134, 17.0975) centre (23.2, 0) ccw projected
  arc A6 (16.4153, 22.8983) -> (18.134, 17.0975) centre (17.2746, 19.9979) ccw projected
  arc A7 (29.9847, 22.8983) -> (16.4153, 22.8983) centre (23.2, 0) ccw projected
  arc A8 (-18.134, 17.0975) -> (-28.266, 17.0975) centre (-23.2, 0) ccw projected
  arc A9 (-29.9847, 22.8983) -> (-28.266, 17.0975) centre (-29.1254, 19.9979) ccw projected
  arc A10 (-16.4153, 22.8983) -> (-29.9847, 22.8983) centre (-23.2, 0) ccw projected
  arc A11 (-18.134, 17.0975) -> (-16.4153, 22.8983) centre (-17.2746, 19.9979) ccw projected
  arc A12 (-16.5766, 26.0535) -> (-30.837, 25.7747) centre (-23.2, 0) ccw projected
  arc A13 (-30.837, 25.7747) -> (-34.5946, 17.4704) centre (-29.1254, 19.9979) ccw projected
  line L4 (-27.4137, -1.5794) -> (-34.5946, 17.4704) projected
  arc A14 (-27.4137, -1.5794) -> (-25.9762, -3.5416) centre (-23.2, 0) ccw projected
  line L5 (-10.0045, -16.0614) -> (-25.9762, -3.5416) projected
  arc A15 (-10.0045, -16.0614) -> (-7.2283, -17.0198) centre (-7.2283, -12.5198) ccw projected
  line L6 (7.2283, -17.0198) -> (-7.2283, -17.0198) projected
  arc A16 (7.2283, -17.0198) -> (10.0045, -16.0614) centre (7.2283, -12.5198) ccw projected
  line L7 (25.9762, -3.5416) -> (10.0045, -16.0614) projected
  arc A17 (25.9762, -3.5416) -> (27.7, 0) centre (23.2, 0) ccw projected
  line L8 (34.7286, 17.7833) -> (27.7, 0) projected
  arc A18 (34.7286, 17.7833) -> (30.837, 25.7747) centre (29.1254, 19.9979) ccw projected
  arc A19 (30.837, 25.7747) -> (16.3694, 26) centre (23.2, 0) ccw projected
  line L9 (-9.4681, 26) -> (16.3694, 26) projected
  circle A20 centre (-23.2, 0) radius 3 projected
  circle A21 centre (23.2, 0) radius 3 projected
  circle A22 centre (-7.2283, -12.5198) radius 3 projected
  circle A23 centre (7.2283, -12.5198) radius 3 projected
  line L10 (0, 0) -> (0, 26)
  line L11 (30.5569, 38.9436) -> (12.9121, 25.6211)
  arc A24 (12.9121, 25.6211) -> (10.2725, 18.6301) centre (17.1301, 20.0347) ccw
  line L12 (10.2725, 18.6301) -> (14.4383, -1.7088)
  arc A25 (14.4383, -1.7088) -> (25.5262, -8.6117) centre (23.2553, 0.0971) ccw
  line L13 (-9.4681, 26) -> (0.0781, 10.7229) projected
  line L14 (-0.3943, 8.6767) -> (-2.964, 7.071) projected
  line L15 (-5.0102, 7.5434) -> (-16.5766, 26.0535) projected
  arc A26 (-0.3943, 8.6767) -> (0.0781, 10.7229) centre (-0.1581, 9.6998) ccw projected
  arc A27 (-5.0102, 7.5434) -> (-2.964, 7.071) centre (-3.9871, 7.3072) ccw projected
  point P0 (13.4139, 26)
  point P1 (23.1707, -5.7407)
  point P2 (-19.9427, -8.2711)
  point P3 (-13.4139, 26)
  point P4 (-31.781, 18.5494)
  point P5 (-14.6743, 21.5435)
  point P6 (21.2542, 26.8118)
  point P7 (-10.7037, 16.5244)
  point P8 (17.3768, 16.9746)
  point P9 (17.6686, 23.2329)
  point P10 (13.4139, 26)
  point P11 (19.9427, -8.2711)
  point P12 (-20.8747, -7.5405)
  point P13 (-19.9427, -8.2711)
  point P14 (-10.6836, 16.6228)
  dimension "d233" = 1
  constraints: 14 end point, 12 point on circle, 7 symmetric about line, 6 centre point, 1 point on line, 1 vertical, 9 other
  measures "d233" distance between parallel lines of L0 L2
extrude "押し出し18" cut sketch "スケッチ17" against normal blind 0.5 contours L15 L3 A3 L5 A1 L1 | L1 A1 L5 A14 L4 A13 A12 L15 | A25 L12 A24 L11 L9 A19 A18 L8 A17 L7 | A5 A6 A7 A4 | A8 A9 A10 A11 | A20
sketch "スケッチ18" plane through (0, 0, 0.5) normal (0, 0, -1) x (-1, 0, 0)
  circle A0 centre (-23.2, 0) radius 3 projected
  circle A1 centre (23.2, 0) radius 3 projected
  circle A2 centre (-23.2, 0) radius 6.025
  circle A3 centre (23.2, 0) radius 6.025
  point P0 (0, 0)
  point P1 (20.2009, -0.0729)
  point P2 (21.187, 2.2244)
  dimension "d236" = 12.05
  dimension "d237" = 12.05
  constraints: 2 centre point, 2 coincident
  measures "d236" diameter of A2
  measures "d237" diameter of A3
extrude "押し出し19" cut sketch "スケッチ18" against normal blind 0.5 contours A1 | A2 | A3
extrude "押し出し21" cut sketch "スケッチ20" against normal blind 2.4 contours A43 A40 A41 L9 A39 L29 A38 L35 | L34 A38 L32 A37 L16 L17 A43 | A38 L25 A36 L11 A35 L23 A46 L15 L31 | L28 A39 L10 A36 L26 A38 | A46 L22 A35 L12 A34 L19 L14 | L20 A34 L13 A33 A30 A31
fillet "フィレット5" radius 1.05 41 edges at (-27.7, 0, 2) (-16.3694, 26, 1.75) (30.9038, 14.767, 1.45) (15.6602, 14.714, 1.45) (21.4702, 5.2209, 1.7) (26.8786, 4.0887, 1.7) (19.3379, 3.9159, 1.7) (20.4016, -4.7348, 1.7) (12.5855, 14.9487, 1.45) (5.681, 3.8992, 1.2) (7.7028, -7.0403, 1.2) (12.4944, -10.933, 1.2) (5.2283, -7.3963, 1.2) (3.9586, 3.5016, 1.2) (2.1048, -14.5198, 1.2) (-2.1048, -14.5198, 1.2) (-6.3602, -7.0887, 1.2) (-5.2934, 4.9759, 1.2) (-6.7643, -1.3868, 1.2) (-8.8885, 6.2684, 1.2) (-7.4565, 6.2293, 1.2) (-11.843, 0.4972, 1.2) (-9.2581, -1.5635, 1.2) (-3.4612, 8.1379, 1.2) (16.5766, 26.0535, 1.75) (9.4681, 26, 1.5) (4.958, 23.5, 1.2) (1.7675, 18.3942, 1.2) (-3.7461, 12.6327, 1.2) (-15.9488, 14.6343, 1.45) (-11.1167, 5.135, 1.2) (-13.0014, 23.5, 1.45) (-13.7205, 15.7678, 1.45) (-30.8398, 14.7456, 1.45) (-12.2263, 2.9676, 1.2) (-18.0989, 2.0564, 1.7) (-26.6914, 4.2497, 1.7) (-17.7156, -0.414, 1.7) (-20.4016, -4.7348, 1.7) (-8.8539, -7.2655, 1.2) (-12.4944, -10.933, 1.2)
chamfer "面取り2" distance 1.5 angle 45 2 edges at (-2.2595, 15.2936, 3) (-9.7799, 2.315, 3)
